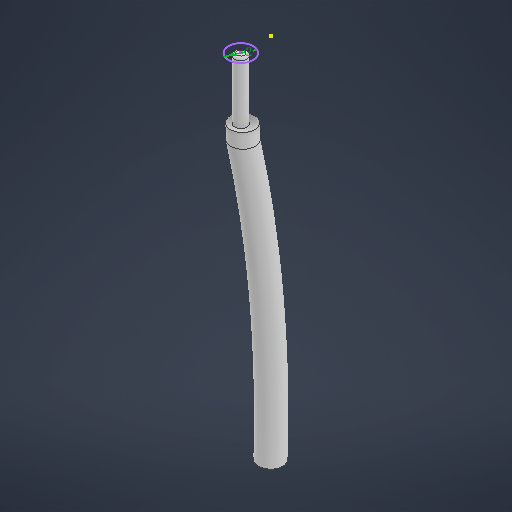
# Autodesk Inventor part: 凸点轴相关
Saved by Autodesk Inventor 2025 (Build 290162000, 162)
## iProperties
Created: 2026-04-16
Part Number: 凸点轴相关
Material: 常规
Document SubType Name: Modeling
Designer: XH
Density: 1 g/cm^3
Appearance: 默认
Author: XH
Autodesk Inventor part; units mm, degrees
ref_plane "YZ Plane" through (0, 0, 0) normal (1, 0, 0) x (0, 1, 0)
ref_plane "XY Plane" through (0, 0, 0) normal (0, 0, 1) x (1, 0, 0)
sketch "草图1" plane through (0, 0, 0) normal (0, 1, 0) x (-1, 0, 0)
  circle A0 centre (0, 0) radius 1
  dimension "d0" = 2
  constraints: 1 centre point, 1 coincident
  measures "d0" diameter of A0
ref_plane "工作平面1" through (0, 30, 0) normal (0, 1, 0) x (-1, 0, 0)
sketch "草图3" plane through (0, 30, 0) normal (0, 1, 0) x (-1, 0, 0)
  circle A0 centre (0, 2.4288) radius 1
  point P0 (0, 0)
  dimension "d8" = 2
  constraints: 1 centre point
  measures "d8" diameter of A0
sketch "草图4" plane through (0, 0, 0) normal (1, 0, 0) x (0, 1, 0)
  arc A0 (0, 0) -> (23.8002, 2.2543) centre (3.1037, 93.9944) ccw
  line L0 (30, 1.4288) -> (30, 3.4288) projected
  line L1 (30, 2.4288) -> (23.8002, 2.2543)
  constraints: 2 end point, 2 point on circle, 1 centre point, 1 midpoint
sweep "扫掠1" add profiles "草图1" path "草图4" keep normal constant yes path curves A0 L1
sketch "草图2" plane through (0, 30, 0) normal (0, 1, 0) x (1, 0, 0)
  circle A0 centre (0, -2.4288) radius 0.5
  circle A1 centre (0, -2.4288) radius 1 projected
  circle A2 centre (0, -2.4288) radius 1 projected
  dimension "d3" = 1
  constraints: 2 coincident, 1 centre point
  measures "d3" diameter of A0
extrude "拉伸2" cut sketch "草图2" against normal blind 5
fillet "圆角1" radius 0.2 1 edges at (-0.5, 30, 2.4288)
delete faces "删除1" heal yes whole lump no faces at (0.9946, 28.3333, 2.325)
